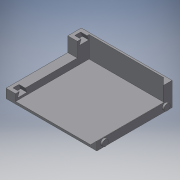
# Autodesk Inventor part: Batcap3
Saved by Autodesk Inventor 2016 SP2 (Build 200236200, 236)
## iProperties
Created: 2018-06-29
Part Number: Batcap3
Material: Generisch
Document SubType Name: Modeling
Designer: Nils
Density: 1 g/cm^3
Appearance: Vorgabe
Author: Nils
Autodesk Inventor part; units mm, degrees
ref_plane "YZ Plane" through (0, 0, 0) normal (1, 0, 0) x (0, 1, 0)
ref_plane "XZ Plane" through (0, 0, 0) normal (0, 1, 0) x (-1, 0, 0)
ref_plane "XY Plane" through (0, 0, 0) normal (0, 0, 1) x (1, 0, 0)
sketch "Skizze1" plane through (0, 0, 0) normal (1, 0, 0) x (0, 1, 0)
  line L0 (12.7735, 187.5054) -> (12.7735, 177.5054) construction
  line L1 (12.7735, 177.5054) -> (95.7735, 177.5054) construction
  line L2 (95.7735, 177.5054) -> (95.7735, 203.5054) construction
  line L3 (91.4537, 203.5054) -> (93.2735, 198.5054) construction
  line L4 (95.7735, 203.5054) -> (80.7735, 203.5054) construction
  line L5 (93.2735, 198.5054) -> (83.2735, 198.5054) construction
  line L6 (83.2735, 198.5054) -> (85.0934, 203.5054) construction
  line L7 (80.7735, 203.5054) -> (80.7735, 187.5054) construction
  line L8 (80.7735, 187.5054) -> (12.7735, 187.5054) construction
  line L9 (12.7735, 187.5054) -> (12.7735, 177.5054) construction
  line L10 (15.2735, 182.5054) -> (17.0934, 187.5054) construction
  line L11 (25.2735, 182.5054) -> (15.2735, 182.5054) construction
  line L12 (23.4537, 187.5054) -> (25.2735, 182.5054) construction
  line L13 (95.7735, 177.5054) -> (95.7735, 203.4054)
  line L14 (95.7735, 203.4054) -> (91.5965, 203.4054)
  line L15 (91.5965, 203.4054) -> (93.4163, 198.4054)
  line L16 (93.4163, 198.4054) -> (83.1307, 198.4054)
  line L17 (83.1307, 198.4054) -> (84.9506, 203.4054)
  line L18 (84.9506, 203.4054) -> (80.8735, 203.4054)
  line L19 (80.8735, 203.4054) -> (80.8735, 187.4054)
  line L20 (80.8735, 187.4054) -> (23.5965, 187.4054)
  line L21 (23.5965, 187.4054) -> (25.4163, 182.4054)
  line L22 (25.4163, 182.4054) -> (15.1307, 182.4054)
  line L23 (15.1307, 182.4054) -> (16.9506, 187.4054)
  line L24 (16.9506, 187.4054) -> (12.8735, 187.4054)
  line L25 (12.8735, 187.4054) -> (12.8735, 177.5054)
  line L26 (12.8735, 177.5054) -> (95.7735, 177.5054)
  point P0 (0, 0)
  dimension "d0" = 0.1
  dimension "d1" = 0.1
  dimension "d2" = 0.1
  dimension "d3" = 0.1
  dimension "d4" = 0.1
  dimension "d5" = 0.1
  dimension "d6" = 0.1
  dimension "d7" = 0.1
  constraints: 28 end point, 15 parallel, 2 point on line, 1 collinear, 1 horizontal, 1 perpendicular
  measures "d0" distance of L2.end L13.end
  measures "d1" distance between parallel lines of L15 L3
  measures "d2" distance between parallel lines of L17 L6
  measures "d3" distance between parallel lines of L19 L7
  measures "d4" distance between parallel lines of L8 L20
  measures "d5" distance between parallel lines of L12 L21
  measures "d6" distance between parallel lines of L10 L23
  measures "d7" distance between parallel lines of L25 L0
extrude "Extrusion1" add sketch "Skizze1" along normal blind 7
sketch "Skizze2" plane through (0, 0, 0) normal (-1, 0, 0) x (0, 0, 1)
  line L0 (177.5054, 95.7735) -> (203.4054, 95.7735) projected
  line L1 (177.5054, 12.8735) -> (177.5054, 95.7735) projected
  line L2 (187.4054, 12.8735) -> (177.5054, 12.8735) projected
  line L3 (203.4054, 80.8735) -> (187.4054, 80.8735) projected
  line L4 (203.4054, 80.8735) -> (187.4054, 80.8735) projected
  line L5 (187.4054, 12.8735) -> (187.4054, 80.8735)
  line L6 (187.4054, 80.8735) -> (203.4054, 80.8735)
  line L7 (203.4054, 95.7735) -> (203.4054, 91.5965) projected
  line L8 (203.4054, 80.8735) -> (203.4054, 95.7735)
  point P0 (0, 0)
  constraints: 6 end point, 1 collinear, 1 perpendicular, 1 vertical
extrude "Extrusion2" add sketch "Skizze2" along normal blind 3.5
sketch "Skizze3" plane through (7, 0, 0) normal (1, 0, 0) x (0, 0, -1)
  line L0 (-177.5054, 95.7735) -> (-203.4054, 95.7735) projected
  line L1 (-177.5054, 12.8735) -> (-177.5054, 95.7735) projected
  line L2 (-177.5054, 12.8735) -> (-180.0054, 12.8735)
  line L3 (-187.4054, 12.8735) -> (-177.5054, 12.8735) projected
  line L4 (-180.0054, 12.8735) -> (-180.0054, 93.7735)
  line L5 (-177.5054, 95.7735) -> (-177.5054, 12.8735) projected
  line L6 (-180.0054, 93.7735) -> (-203.4054, 93.7735)
  line L7 (-203.4054, 95.7735) -> (-203.4054, 91.5965) projected
  line L8 (-203.4054, 93.7735) -> (-203.4054, 95.7735)
  point P0 (0, 0)
  dimension "d12" = 2.5
  dimension "d13" = 2
  dimension "d14" = 2
  constraints: 8 end point, 1 parallel, 1 perpendicular, 1 point on line
  measures "d12" distance of L1.start L2.end
  measures "d13" distance from line of L0 L4.end
  measures "d14" distance of L0.end L6.end
extrude "Extrusion3" add sketch "Skizze3" along normal blind 89.5
sketch "Skizze4" plane through (96.5, 0, 0) normal (1, 0, 0) x (0, 0, -1)
  circle A0 centre (-182.5054, 20.2735) radius 3.5 construction
  circle A1 centre (-182.5054, 88.2735) radius 3.5 construction
  circle A2 centre (-182.5054, 20.2735) radius 3.45
  circle A3 centre (-182.5054, 88.2735) radius 3.45
  point P0 (0, 0)
  dimension "d17" = 0.05
  dimension "d18" = 0.05
  constraints: 2 centre point
  measures "d17" radial gap between concentric circles of A0 A2
  measures "d18" radial gap between concentric circles of A1 A3
extrude "Extrusion4" add sketch "Skizze4" along normal blind 2
sketch "Skizze5" plane through (96.5, 0, 0) normal (1, 0, 0) x (0, 0, -1)
  line L0 (-198.9754, 90.3435) -> (-183.0054, 90.3435) construction
  line L1 (-180.0054, 17.896) -> (-180.0054, 12.8735) projected
  circle A0 centre (-182.5054, 88.2735) radius 3.5 construction
  line L2 (-203.4054, 93.7735) -> (-180.0054, 93.7735) projected
  line L3 (-180.0054, 12.8735) -> (-186.5054, 12.8735)
  line L4 (-186.5054, 12.8735) -> (-186.5054, 93.7735)
  line L5 (-186.5054, 93.7735) -> (-180.0054, 93.7735)
  line L6 (-180.0054, 93.7735) -> (-180.0054, 12.8735)
  line L7 (-203.4054, 93.7735) -> (-186.5054, 93.7735)
  line L8 (-186.5054, 93.7735) -> (-186.5054, 86.7735)
  line L9 (-186.5054, 86.7735) -> (-203.4054, 86.7735)
  line L10 (-203.4054, 86.7735) -> (-203.4054, 93.7735)
  point P0 (0, 0)
  point P1 (-186.5054, 90.3435)
  dimension "d27" = 4
  dimension "d31" = 7
  constraints: 16 end point, 4 parallel, 3 point on line, 2 horizontal, 2 perpendicular
  measures "d27" distance from line of L4 A0.centre
  measures "d31" distance of L7.end L8.end
extrude "Extrusion5" add sketch "Skizze5" against normal blind 7
chamfer "Fase2" distance 6.5 angle 45 1 edges at (89.5, 49.8235, 186.5054)
chamfer "Fase3" distance 6.5 angle 45 1 edges at (89.5, 86.7735, 194.9554)
equation "\"d14\" = d13"
